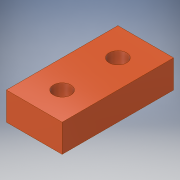
# Autodesk Inventor part: seatingPartsExample
Saved by Autodesk Inventor 2019.3 (Build 233278000, 278)
## iProperties
Created: 2019-01-12
Part Number: seatingPartsExample
Material: Phenolic Resin
Document SubType Name: Modeling
Designer: steele
Density: 1.38 g/cm^3
Appearance: Smooth - Light Orange
Author: steele
Autodesk Inventor part; units mm, degrees
ref_plane "YZ Plane" through (0, 0, 0) normal (1, 0, 0) x (0, 1, 0)
ref_plane "XZ Plane" through (0, 0, 0) normal (0, 1, 0) x (-1, 0, 0)
ref_plane "XY Plane" through (0, 0, 0) normal (0, 0, 1) x (1, 0, 0)
sketch "Sketch1" plane through (0, 0, 0) normal (0, 0, 1) x (1, 0, 0)
  line L0 (-12.7, -6.35) -> (12.7, -6.35)
  line L1 (12.7, -6.35) -> (12.7, 6.35)
  line L2 (12.7, 6.35) -> (-12.7, 6.35)
  line L3 (-12.7, 6.35) -> (-12.7, -6.35)
  line L4 (-12.7, -6.35) -> (12.7, 6.35) construction
  line L5 (12.7, -6.35) -> (-12.7, 6.35) construction
  point P0 (0, 0)
  dimension "d0" = 25.4
  dimension "d1" = 12.7
  constraints: 12 end point, 2 midpoint, 2 parallel, 1 horizontal, 1 perpendicular
  measures "d0" distance of L0.start L0.end
  measures "d1" distance of L1.end L0.end
extrude "Extrusion1" add sketch "Sketch1" along normal mid plane 50.8
sketch "Sketch2" plane through (-12.7, 6.35, 25.4) normal (0, 1, 0) x (1, 0, 0)
  line L0 (25.4, 0) -> (0, 0) projected
  line L1 (0, 50.8) -> (25.4, 50.8) projected
  point P0 (12.7, 25.4)
  point P1 (12.7, 12.7)
  point P2 (12.7, 38.1)
  dimension "d11" = 12.7
  dimension "d12" = 12.7
  measures "d11" distance from line of point (12.7, 12.7) L0
  measures "d12" distance from line of point (12.7, 38.1) L1
hole "Hole1" at (0, 6.35, 12.7) at (0, 6.35, -12.7) direction (0, -1, 0) diameter 6.7564 end through all counterbore diameter 8.0264 counterbore depth 9.525 clearance for "Hex Head Bolt" size "1/4" standard "Ansi Unified Screw Threads"
body "Solid1"
